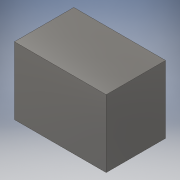
# Autodesk Inventor part: PiEthernet
Saved by Autodesk Inventor 2018 (Build 220112000, 112)
## iProperties
Created: 2018-01-13
Part Number: PiEthernet
Material: Stainless Steel
Document SubType Name: Modeling
Designer: Kyle-HP
Density: 8 g/cm^3
Appearance: Semi-Polished
Author: Kyle-HP
Autodesk Inventor part; units mm, degrees
ref_plane "YZ Plane" through (0, 0, 0) normal (1, 0, 0) x (0, 1, 0)
ref_plane "XZ Plane" through (0, 0, 0) normal (0, 1, 0) x (-1, 0, 0)
ref_plane "XY Plane" through (0, 0, 0) normal (0, 0, 1) x (1, 0, 0)
sketch "Sketch1" plane through (0, 0, 0) normal (0, 0, 1) x (1, 0, 0)
  line L0 (0, 0) -> (21.59, 0)
  line L1 (21.59, 0) -> (21.59, -15.875)
  line L2 (21.59, -15.875) -> (0, -15.875)
  line L3 (0, -15.875) -> (0, 0)
  dimension "d0" = 21.59
  dimension "d1" = 15.875
  constraints: 8 end point, 2 parallel, 1 horizontal, 1 perpendicular
  measures "d0" distance of L0.start L0.end
  measures "d1" distance of L0.end L1.end
extrude "Extrusion1" add sketch "Sketch1" along normal blind 13.97
body "Solid1"
